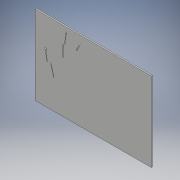
# Autodesk Inventor part: metacarpus geometry
Saved by Autodesk Inventor 2017 (Build 210142000, 142)
## iProperties
Created: 2018-01-25
Part Number: metacarpus geometry
Material: Generic
Document SubType Name: Modeling
Designer: Tomasz
Density: 1 g/cm^3
Appearance: Default
Author: Tomasz
Autodesk Inventor part; units mm, degrees
ref_plane "YZ Plane" through (0, 0, 0) normal (1, 0, 0) x (0, 1, 0)
ref_plane "XZ Plane" through (0, 0, 0) normal (0, 1, 0) x (-1, 0, 0)
sketch "Sketch2" plane through (0, 0, 0) normal (0, 1, 0) x (-1, 0, 0)
  line L0 (0, 0) -> (220, 0)
  line L1 (220, 0) -> (220, -150)
  line L2 (220, -150) -> (0, -150)
  line L3 (0, -150) -> (0, 0)
  dimension "d0" = 150
  dimension "d1" = 220
  constraints: 8 end point, 2 parallel, 1 horizontal, 1 perpendicular
  measures "d0" distance of L0.end L1.end
  measures "d1" distance of L1.end L2.end
extrude "Plate" add sketch "Sketch2" along normal blind 2
sketch "Sketch3" plane through (0, 2, 0) normal (0, 1, 0) x (1, 0, 0)
  point P0 (0, 0)
  point P1 (-161, 10)
  dimension "d4" = 161
  dimension "d5" = 10
  measures "d4" horizontal distance of point (-161, 10) point (0, 0)
  measures "d5" vertical distance of point (-161, 10) point (0, 0)
hole "Finger 2 position" at (-161, 2, -10) direction (0, -1, 0) diameter 3 end through all
sketch "Sketch4" plane through (0, 2, 0) normal (0, 1, 0) x (1, 0, 0)
  circle A0 centre (-161, 10) radius 1.5 projected
  line L0 (-161, 10) -> (-164.1646, 32.5171) construction
  line L1 (-161, 10) -> (-161, 35.4885) construction
  line L2 (-161.4951, 9.9304) -> (-161, 10)
  line L3 (-161, 10) -> (-160.5049, 10.0696)
  line L4 (-161.4951, 9.9304) -> (-164.2786, 29.7358)
  line L5 (-164.2786, 29.7358) -> (-163.2883, 29.8749)
  line L6 (-163.2883, 29.8749) -> (-160.5049, 10.0696)
  point P0 (0, 0)
  dimension "d14" = 1
  dimension "d15" = 20
  dimension "d32" = 8
  constraints: 14 end point, 2 perpendicular, 1 parallel, 1 point on line, 1 vertical, 1 other
  measures "d14" distance between parallel lines of L6 L4
  measures "d15" distance between parallel lines of L2 L5
  measures "d32" angle of L0 L1
extrude "Finger 2 angle" cut sketch "Sketch4" against normal through all contours L6 L3 L2 L4 A0 | A0 L4 L5 L6 picked at (-161.3957, 10.4204)
sketch "Sketch5" plane through (0, 2, 0) normal (0, 1, 0) x (1, 0, 0)
  point P0 (0, 0)
  point P1 (-167, 33)
  dimension "d18" = 33
  dimension "d19" = 167
  measures "d18" vertical distance of point (-167, 33) point (0, 0)
  measures "d19" horizontal distance of point (-167, 33) point (0, 0)
hole "Finger 3 position" at (-167, 2, -33) direction (0, -1, 0) diameter 3 end through all
sketch "Sketch6" plane through (0, 2, 0) normal (0, 1, 0) x (1, 0, 0)
  circle A0 centre (-167, 33) radius 1.5 projected
  line L0 (-167, 33) -> (-167, 67.5) construction
  line L1 (-167, 33) -> (-167, 65.8824) construction
  line L2 (-167.5, 33) -> (-167, 33)
  line L3 (-167, 33) -> (-166.5, 33)
  line L4 (-167.5, 33) -> (-167.5, 53)
  line L5 (-167.5, 53) -> (-166.5, 53)
  line L6 (-166.5, 53) -> (-166.5, 33)
  point P0 (0, 0)
  dimension "d27" = 0
  dimension "d28" = 1
  dimension "d29" = 20
  constraints: 14 end point, 3 perpendicular, 1 point on line, 1 vertical, 1 other
  measures "d27" distance between parallel lines of L1 L0
  measures "d28" distance between parallel lines of L6 L4
  measures "d29" distance between parallel lines of L5 L2
extrude "Finger 3 angle" cut sketch "Sketch6" against normal through all contours L6 L3 L2 L4 A0 | A0 L4 L5 L6 picked at (-167.3333, 33.4714)
sketch3d "Thumb joint geometry"
ref_plane "Work Plane1" through (-129.5, -9.5, -13) normal (0.8447, 0.4001, -0.3556) x (-0.4281, 0.9037, 0)
sketch "Sketch7" plane through (-129.5, -9.5, -13) normal (0.8447, 0.4001, -0.3556) x (-0.4281, 0.9037, 0)
  circle A0 centre (0, 0) radius 5
  point P0 (-46.8517, 55.2188)
  dimension "d39" = 10
  constraints: 1 centre point, 1 coincident
  measures "d39" diameter of A0
extrude "Thumb joint" add sketch "Sketch7" along normal blind 1
sketch "Sketch9" plane through (0, 2, 0) normal (0, 1, 0) x (1, 0, 0)
  circle A0 centre (-200, 55) radius 1.5
  line L0 (-196.7214, 74.7358) -> (-199.5049, 54.9304)
  line L1 (-199.5049, 54.9304) -> (-200.4951, 55.0696)
  line L2 (-200.4951, 55.0696) -> (-197.7117, 74.8749)
  line L3 (-197.7117, 74.8749) -> (-196.7214, 74.7358)
  line L4 (-196.7214, 74.7358) -> (-200.4951, 55.0696) construction
  line L5 (-199.5049, 54.9304) -> (-197.7117, 74.8749) construction
  line L6 (-200, 55) -> (-92.8888, 55) construction
  point P0 (0, 0)
  point P1 (-198.6083, 64.9027)
  dimension "d42" = 20
  dimension "d43" = 3
  dimension "d44" = 200
  dimension "d45" = 55
  dimension "d47" = 82
  dimension "d48" = 1
  constraints: 14 end point, 3 midpoint, 2 parallel, 1 centre point, 1 horizontal, 1 perpendicular
  measures "d42" distance of L1.end L2.end
  measures "d43" diameter of A0
  measures "d44" horizontal distance of L6.start point (0, 0)
  measures "d45" vertical distance of point (0, 0) L6.start
  measures "d47" angle of L0 L6
  measures "d48" distance between parallel lines of L0 L2
extrude "Finger 3" cut sketch "Sketch9" against normal through all
sketch "Sketch10" plane through (0, 2, 0) normal (0, 1, 0) x (1, 0, 0)
  circle A0 centre (-190, 75) radius 1.5
  line L0 (-184.0066, 94.0874) -> (-189.5194, 74.8622)
  line L1 (-189.5194, 74.8622) -> (-190.4806, 75.1378)
  line L2 (-190.4806, 75.1378) -> (-184.9679, 94.3631)
  line L3 (-184.9679, 94.3631) -> (-184.0066, 94.0874)
  line L4 (-184.0066, 94.0874) -> (-190.4806, 75.1378) construction
  line L5 (-189.5194, 74.8622) -> (-184.9679, 94.3631) construction
  line L6 (-190, 75) -> (-75.9657, 75) construction
  point P0 (0, 0)
  point P1 (-187.2436, 84.6126)
  dimension "d51" = 3
  dimension "d52" = 1
  dimension "d53" = 20
  dimension "d54" = 190
  dimension "d55" = 75
  dimension "d56" = 74
  constraints: 14 end point, 3 midpoint, 2 parallel, 1 centre point, 1 horizontal, 1 perpendicular
  measures "d51" diameter of A0
  measures "d52" distance between parallel lines of L0 L2
  measures "d53" distance from line of L6.start L3
  measures "d54" horizontal distance of point (0, 0) L6.start
  measures "d55" vertical distance of L6.start point (0, 0)
  measures "d56" angle of L0 L6
extrude "Finger 4" cut sketch "Sketch10" against normal through all
equation "\"d4\" = finger_2_z"
equation "\"d5\" = finger_2_x"
equation "\"d32\" = finger_2_angle"
equation "\"d18\" = finger_3_x"
equation "\"d19\" = finger_3_z"
equation "\"d33\" = thumb_CMC_x"
equation "\"d34\" = thumb_CMC_z"
equation "\"d35\" = thumb_CMC_y"
equation "\"d36\" = thumb_CMC_axis_z"
equation "\"d37\" = -thumb_CMC_axis_x"
equation "\"d38\" = thumb_CMC_axis_y"
equation "\"d44\" = finger_4_x"
equation "\"d45\" = finger_4_z"
equation "\"d54\" = finger_5_x"
equation "\"d55\" = finger_5_z"
equation "\"thumb_CMC_axis_x\" = thumb_axis_x"
equation "\"thumb_CMC_axis_y\" = thumb_axis_y"
equation "\"thumb_CMC_axis_z\" = thumb_axis_z"
equation "\"thumb_CMC_x\" = thumb_x"
equation "\"thumb_CMC_y\" = thumb_y"
equation "\"finger_2_x\" = F2_x"
equation "\"finger_2_z\" = F2_z"
equation "\"finger_2_angle\" = F2_angle"
equation "\"finger_3_x\" = F3_x"
equation "\"finger_3_z\" = F3_z"
equation "\"finger_4_x\" = F4_x"
equation "\"finger_4_z\" = F4_z"
equation "\"finger_4_angle\" = F4_angle"
equation "\"finger_5_x\" = F5_x"
equation "\"finger_5_z\" = F5_z"
equation "\"finger_5_angle\" = F5_angle"
equation "\"thumb_CMC_z\" = 120"
equation "\"thumb_axis_x\" = -0.4"
equation "\"thumb_axis_y\" = 0.45"
equation "\"thumb_axis_z\" = 0.95"
equation "\"thumb_x\" = 17"
equation "\"thumb_y\" = 5"
equation "\"F2_x\" = 10"
equation "\"F2_z\" = 161"
equation "\"F2_angle\" = 8deg"
equation "\"F3_x\" = 33"
equation "\"F3_z\" = 167"
equation "\"F4_x\" = 200"
equation "\"F4_z\" = 55"
equation "\"F4_angle\" = -8deg"
equation "\"F5_x\" = 190"
equation "\"F5_z\" = 75"
equation "\"F5_angle\" = -16deg"
body "Solid1"
